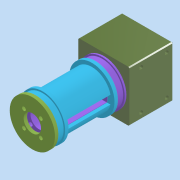
# Autodesk Inventor part: ForearmShaft2
Saved by Autodesk Inventor 2020.2 (Build 242310000, 310)
## iProperties
Created: 2020-02-16
Part Number: ForearmShaft2
Material: Generisch
Document SubType Name: Modeling
Designer: JochenAlt
Density: 1 g/cm^3
Appearance: Vorgabe
Author: JochenAlt
Autodesk Inventor part; units mm, degrees
ref_plane "YZ Plane" through (0, 0, 0) normal (1, 0, 0) x (0, 1, 0)
ref_plane "XZ Plane" through (0, 0, 0) normal (0, 1, 0) x (-1, 0, 0)
ref_plane "XY Plane" through (0, 0, 0) normal (0, 0, 1) x (1, 0, 0)
sketch "Main" plane through (0, 0, 0) normal (0, 0, 1) x (1, 0, 0)
  line L0 (0, 37.6444) -> (0, -28.4407) construction
  line L1 (-34.1979, 0) -> (72.1871, 0) construction
  line L2 (0, -28.4407) -> (0, 37.6444) construction
  line L3 (-34.1979, 0) -> (72.1871, 0) construction
  circle A0 centre (0, 0) radius 19 construction
  line L4 (-19, 0) -> (-9.5, 16.4545) construction
  line L5 (-9.5, 16.4545) -> (9.5, 16.4545) construction
  line L6 (9.5, 16.4545) -> (19, 0) construction
  line L7 (19, 0) -> (9.5, -16.4545) construction
  line L8 (9.5, -16.4545) -> (-9.5, -16.4545) construction
  line L9 (-9.5, -16.4545) -> (-19, 0) construction
  arc A1 (-12.8789, -3.3204) -> (-9.6592, -9.1427) centre (0, 0) ccw
  circle A2 centre (0, 0) radius 13.3
  circle A3 centre (0, 0) radius 7 construction
  circle A4 centre (0, 0) radius 17 construction
  circle A5 centre (0, 0) radius 5.1
  circle A6 centre (-4.9497, -4.9497) radius 1.1
  circle A7 centre (4.9497, -4.9497) radius 1.1
  circle A8 centre (4.9497, 4.9497) radius 1.1
  circle A9 centre (-4.9497, 4.9497) radius 1.1
  circle A10 centre (0, 0) radius 9
  circle A11 centre (0, 0) radius 12.4
  circle A12 centre (0, 0) radius 9.2
  circle A13 centre (0, 0) radius 11.2
  line L10 (15, 15) -> (-15, 15)
  line L11 (-15, 15) -> (-15, -15)
  line L12 (-15, -15) -> (15, -15)
  line L13 (15, -15) -> (15, 15)
  line L14 (-4.9497, -4.9497) -> (4.9497, -4.9497) construction
  line L15 (4.9497, -4.9497) -> (4.9497, 4.9497) construction
  line L16 (-4.9497, 4.9497) -> (-4.9497, -4.9497) construction
  line L17 (-4.9497, 4.9497) -> (4.9497, 4.9497) construction
  point P0 (9.5, -16.4545)
  point P1 (9.5, 16.4545)
  point P2 (37.0107, 21.6054)
  point P3 (37.0107, 13.3946)
  point P4 (45.5607, 6.7963)
  point P5 (48.4393, 6.7963)
  point P6 (55.55, 10.9017)
  point P7 (56.9893, 13.3946)
  point P8 (56.9893, 21.6054)
  point P9 (55.55, 24.0983)
  point P10 (48.4393, 28.2037)
  point P11 (45.5607, 28.2037)
  point P12 (38.45, 24.0983)
  point P13 (-12.8789, -3.3204)
  point P14 (-4.1132, 5.664)
  point P15 (4.1132, 5.664)
  point P16 (5.664, 4.1132)
  point P17 (-4.1132, -5.664)
  point P18 (-5.664, -4.1132)
  point P19 (-5.664, 4.1132)
  dimension "d79" = 26.6
  dimension "d28" = 38
  dimension "d31" = 14
  dimension "d41" = 2.2
  dimension "d42" = 2
  dimension "d43" = 10.2
  dimension "d52" = 0.2
  dimension "d67" = 24.8
  dimension "d77" = 2
  dimension "d78" = 30
  constraints: 28 end point, 13 centre point, 11 coincident, 9 point on circle, 5 perpendicular, 3 equal radius, 3 parallel, 3 point on line, 1 horizontal, 18 other
  measures "d28" diameter of A0
  measures "d31" diameter of A3
  measures "d41" diameter of A6
  measures "d42" radial gap between concentric circles of A3 A10
  measures "d43" diameter of A5
  measures "d52" radial gap between concentric circles of A12 A10
  measures "d67" diameter of A11
  measures "d77" radial gap between concentric circles of A13 A12
  measures "d78" distance of L10.end L11.end
extrude "Extrusion21" add sketch "Main" along normal blind 25.8 contours A2 A1 | A10 | A11 | A12 | A13 | L13 L12 L11 L10
extrude "Extrusion22" cut sketch "Main" along normal blind 5 contours A6 | A7 | A8 | A9 | A10
extrude "Extrusion11" add sketch "Main" along normal blind 1 from surface at 25.8 separate body contours A2 A1 | A10 | A11 | A12 | A13
extrude "Extrusion13" add sketch "Main" along normal blind 4 from surface at 26.8 contours A10 | A11 | A12 | A13 bodies 2
extrude "Extrusion14" add sketch "Main" along normal blind 33 from surface at 30.8 contours A10 bodies 2
extrude "Extrusion15" add sketch "Main" along normal blind 31 from surface at 30.8 separate body contours A2 A1 | A11 | A13
extrude "Extrusion16" add sketch "Main" along normal blind 4 from surface at 61.8 contours A11 | A13 bodies 3
extrude "Extrusion17" add sketch "Main" along normal blind 2 from surface at 65.8 separate body contours A2 A1 | A10 | A11 | A12 | A13
ref_plane "Arbeitsebene3" through (0, 0, 59.8) normal (0, 0, 1) x (1, 0, 0)
sketch "Skizze3" plane through (0, 0, 59.8) normal (0, 0, -1) x (-1, 0, 0)
  circle A0 centre (0, 0) radius 5 construction
  line L0 (-13.0629, 2.5) -> (-4.3301, 2.5)
  line L1 (-4.3301, -2.5) -> (-13.0629, -2.5)
  line L2 (0, 0) -> (-13.3, 0) construction
  line L3 (0, 0) -> (13.3, 0) construction
  arc A1 (-4.3301, 2.5) -> (-4.3301, -2.5) centre (0, 0) ccw
  arc A2 (-13.0629, 2.5) -> (-13.0629, -2.5) centre (0, 0) ccw
  circle A3 centre (0, 0) radius 13.3 construction
  dimension "d62" = 180
  dimension "d63" = 5
  dimension "d93" = 10
  constraints: 8 end point, 7 point on circle, 4 coincident, 3 centre point, 1 collinear, 1 horizontal, 1 parallel, 3 other
  measures "d62" angle of L3 L2
  measures "d63" distance between parallel lines of L1 L0
  measures "d93" diameter of A0
extrude "Extrusion19" cut sketch "Skizze3" along normal blind 27 bodies 3 2
extrude "Extrusion20" cut sketch "Main" against normal up to surface (27 mm away) from surface at 59.8 contours A2 A1 | A11 bodies 3
sketch "Skizze4" plane through (0, 0, 0) normal (1, 0, 0) x (0, 1, 0)
  line L0 (-11.5, 18.8) -> (11.5, 18.8) construction
  line L1 (11.5, 18.8) -> (11.5, 3.8) construction
  line L2 (11.5, 3.8) -> (-11.5, 3.8) construction
  line L3 (-11.5, 3.8) -> (-11.5, 18.8) construction
  line L4 (0, -4.96) -> (0, 29.76) construction
  line L5 (-15, 0) -> (15, 0) construction
  circle A0 centre (-11.5, 18.8) radius 1.1
  circle A1 centre (-11.5, 3.8) radius 1.1
  circle A2 centre (11.5, 3.8) radius 1.1
  circle A3 centre (11.5, 18.8) radius 1.1
  point P0 (0, 0)
  point P1 (15, 25.8)
  dimension "d84" = 23
  dimension "d85" = 15
  dimension "d87" = 2.2
  dimension "d94" = 7
  constraints: 8 end point, 4 centre point, 4 coincident, 3 equal radius, 2 parallel, 1 horizontal, 1 perpendicular, 1 other
  measures "d84" distance of L1.end L2.end
  measures "d85" distance of L2.end L0.start
  measures "d87" diameter of A0
  measures "d94" distance from line of point (15, 25.8) L0
extrude "Extrusion23" cut sketch "Skizze4" along normal through all both and the other way through all bodies 1
chamfer "Fase3" distance 0.5 angle 45 8 edges at (15, 15, 12.9) (-15, 15, 12.9) (15, -15, 12.9) (-15, -15, 12.9) (0, -15, 0) (0, 15, 0) (-15, 0, 0) (15, 0, 0)
sketch "Skizze5" plane through (0, 0, 0) normal (0, 0, -1) x (-1, 0, 0)
  circle A0 centre (0, 0) radius 9 construction
  line L0 (0, 4) -> (15, 4)
  line L1 (15, 4) -> (15, -4)
  line L2 (15, -4) -> (0, -4)
  line L3 (0, -4) -> (0, 4)
  line L4 (21, 0) -> (-21, 0) construction
  line L5 (0, -21) -> (0, 21) construction
  line L6 (15, -14.5) -> (15, 14.5) construction
  line L7 (15, 14.5) -> (15, -14.5) construction
  line L8 (15, -10.4) -> (15, -12.6) construction
  line L9 (15, 12.6) -> (15, 10.4) construction
  line L10 (15, -10.4) -> (15, -12.6) construction
  line L11 (15, 12.6) -> (15, 10.4) construction
  point P0 (0, 0)
  dimension "d98" = 8
  constraints: 8 end point, 2 perpendicular, 1 collinear, 1 horizontal, 1 point on line, 1 other
  measures "d98" distance of L0.end L1.end
extrude "Extrusion24" cut sketch "Skizze5" against normal blind 1 bodies 1
fillet "Rundung3" radius 2 1 edges at (-9, 0, 1)
equation "\"d52\" = tight_fit"
equation "\"roundness_small\" = 3"
equation "\"roundness_tiny\" = 0.5"
equation "\"wall_thickness\" = 3"
equation "\"medium_arm_width\" = 51"
equation "\"big_arm_width\" = 56"
equation "\"bevel_angle\" = 20deg"
equation "\"medium_arm_radius\" = 35"
equation "\"big_arm_radius\" = 48"
equation "\"medium_arm_circle_centre\" = 11"
equation "\"big_arm_circle_centre\" = 25"
equation "\"thickness\" = 3"
equation "\"tight_fit\" = 0.2"
equation "\"press_fit\" = 0.1"
equation "\"m2_hex_width\" = 4.2"
equation "\"m2_washer_diameter\" = 5.2"
equation "\"m2_screw_hole_diameter\" = 2.2"
equation "\"m2_allen_screw_width\" = 4"
equation "\"m2_allen_screw_height\" = 2"
equation "\"m2_washer_height\" = 0.3"
